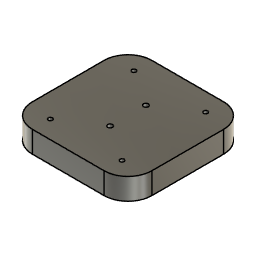
case_rain (Autodesk Fusion 360 design; units mm, degrees)
Autodesk Fusion 360 part; units mm, degrees
sketch "Sketch1" plane through (0, 0, 0) normal (0, 0, 1) x (1, 0, 0)
  line L0 (50, 50) -> (-50, 50)
  line L1 (-50, 50) -> (-50, -50)
  line L2 (-50, -50) -> (50, -50)
  line L3 (50, -50) -> (50, 50)
  line L4 (50, 50) -> (-50, -50) construction
  line L5 (-50, 50) -> (50, -50) construction
  circle A0 centre (0, 15) radius 2.05
  circle A1 centre (0, -15) radius 2.05
  circle A2 centre (0, 15) radius 4
  circle A3 centre (0, -15) radius 4
  circle A4 centre (30, -35) radius 1.75
  circle A5 centre (30, 35) radius 1.75
  line L6 (0, 0) -> (0, 5)
  circle A6 centre (-30, 35) radius 1.75
  circle A7 centre (-30, -35) radius 1.75
  dimension "d1" = 100
  dimension "d2" = 100
  dimension "d4" = 4.1
  dimension "d5" = 15
  dimension "d6" = 15
  dimension "d8" = 8
  dimension "d36" = 3.5
  dimension "d37" = 3.5
  dimension "d55" = 30
  dimension "d56" = 35
  dimension "d57" = 35
  dimension "d58" = 30
  constraint horizontal L0
  constraint perpendicular L0 L1
  constraint parallel L0 L2
  constraint parallel L1 L3
  constraint coincident L4 L6.start
  constraint coincident L5 L6.start
  constraint coincident L6.start origin
  constraint concentric A0 A2
  constraint concentric A1 A3
  constraint vertical L6
  constraint symmetric A4 L6 A7
  constraint symmetric A5 L6 A6
  constraint equal A0 A1
  constraint equal A2 A3
  constraint vertical L6.start A1.centre
  constraint vertical L6.start A0.centre
  measures "d1" distance of L1.end L2.end
  measures "d2" distance of L0.end L1.end
  measures "d4" diameter of A1
  measures "d5" distance of L6.start A0.centre
  measures "d6" distance of L6.start A1.centre
  measures "d8" diameter of A3
  measures "d36" diameter of A4
  measures "d37" diameter of A5
  measures "d55" horizontal distance of L6.start A5.centre
  measures "d56" vertical distance of L6.start A5.centre
  measures "d57" vertical distance of L6.start A4.centre
  measures "d58" horizontal distance of L6.start A4.centre
extrude "Extrude1" add sketch "Sketch1" along normal blind 3 contours L0 L1 L2 L3 | A2 | A3
extrude "Extrude2" add sketch "Sketch1" against normal blind 5 contours A2 | A3
sketch "Sketch2" plane through (0, 0, -5) normal (0, 0, -1) x (1, 0, 0)
  circle A0 centre (0, 15) radius 2.05
  circle A1 centre (0, 15) radius 4
  circle A2 centre (0, 15) radius 3
  circle A3 centre (0, -15) radius 4
  dimension "d40" = 8
  constraint concentric A0 A2
  measures "d40" diameter of A3
extrude "Extrude3" add sketch "Sketch2" along normal blind 2 contours A0 | A1 | A2 | A3
sketch "Sketch3" plane through (0, 0, 0) normal (0, 0, -1) x (1, 0, 0)
  circle A0 centre (0, -15) radius 4
  circle A1 centre (0, 15) radius 4
  line L0 (50, -50) -> (50, 50)
  line L1 (50, 50) -> (-50, 50)
  line L2 (-50, 50) -> (-50, -50)
  line L3 (-50, -50) -> (50, -50)
  circle A2 centre (30, 35) radius 1.75
  circle A3 centre (30, -35) radius 1.75
  line L4 (-47, 42) -> (47, 42)
  line L5 (47, 42) -> (47, -42)
  line L6 (47, -42) -> (-47, -42)
  line L7 (-47, -42) -> (-47, 42)
  circle A4 centre (-30, 35) radius 1.75
  circle A5 centre (-30, -35) radius 1.75
  dimension "d41" = 3
  dimension "d42" = 3
  dimension "d43" = 8
  dimension "d44" = 8
  constraint horizontal L4
  constraint vertical L5
  constraint horizontal L6
  constraint vertical L7
  measures "d41" distance of L0 L5
  measures "d42" distance of L2 L7
  measures "d43" distance of L3 L6
  measures "d44" distance of L1 L4
extrude "Extrude4" add sketch "Sketch3" along normal blind 15 contours L0 L1 L2 L3
sketch "Sketch6" plane through (0, 0, -15) normal (0, 0, -1) x (1, 0, 0)
  line L0 (47, -42) -> (-47, -42)
  line L1 (-47, -42) -> (-47, 42)
  line L2 (-47, 42) -> (47, 42)
  line L3 (47, 42) -> (47, -42)
  line L4 (-50, -50) -> (50, -50)
  line L5 (50, -50) -> (50, 50)
  line L6 (50, 50) -> (-50, 50)
  line L7 (-50, 50) -> (-50, -50)
  line L8 (0, 0) -> (20, 0)
  circle A0 centre (10, 46) radius 2.05
  line L9 (0, 0) -> (0, 5)
  circle A1 centre (-10, 46) radius 2.05
  circle A2 centre (10, -46) radius 2.05
  circle A3 centre (-10, -46) radius 2.05
  dimension "d45" = 4.1
  dimension "d61" = 4
  dimension "d62" = 10
  constraint coincident L8.start L9.start
  constraint parallel L2 L8
  constraint perpendicular L8 L9
  constraint symmetric A0 L9 A1
  constraint symmetric L8 A0 A2
  constraint symmetric L8 A1 A3
  measures "d45" diameter of A0
  measures "d61" distance of L6 A0.centre
  measures "d62" distance of A0.centre L9
extrude "Extrude7" cut sketch "Sketch6" against normal blind 10 contours A0 | A1 | A2 | A3
fillet "Fillet3" radius 20 8 edges at (47, -42, -7.5) (47, 42, -7.5) (-47, -42, -7.5) (50, -50, -6) (-50, -50, -6) (-50, 50, -6) (-47, 42, -7.5) (50, 50, -6)
